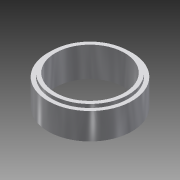
# Autodesk Inventor part: Aluminum Retainer
Saved by Autodesk Inventor 2015 (Build 190159000, 159)
## iProperties
Created: 2016-01-09
Part Number: Aluminum Retainer
Material: Aluminum 6061-AHC
Document SubType Name: Modeling
Designer: Jared
Density: 2.7 g/cm^3
Appearance: Aluminum - Dark
Author: Jared
Autodesk Inventor part; units mm, degrees
ref_plane "YZ Plane" through (0, 0, 0) normal (1, 0, 0) x (0, 1, 0)
ref_plane "XZ Plane" through (0, 0, 0) normal (0, 1, 0) x (-1, 0, 0)
ref_plane "XY Plane" through (0, 0, 0) normal (0, 0, 1) x (1, 0, 0)
sketch "Sketch1" plane through (0, 0, 0) normal (0, 0, 1) x (1, 0, 0)
  arc A0 (-19.4827, -3.287) -> (-19.05, 0) centre (-31.75, 0) ccw
  line L0 (-19.4827, -3.287) -> (-58.7375, -149.7878)
  line L1 (-65.8876, 46.8376) -> (-65.8876, 21.4376)
  line L2 (-65.8876, 21.4376) -> (-71.4375, 21.4376)
  arc A1 (-19.05, 0) -> (-65.8876, 46.8376) centre (-65.8876, 0) ccw
  line L3 (-44.45, 34.1376) -> (-33.8192, 34.1376)
  line L4 (-44.45, 34.1376) -> (-37.3992, -46.4536)
  line L5 (-44.45, 34.1376) -> (0, 34.1376) construction
  line L6 (-37.3992, -46.4536) -> (-31.0492, -46.4536)
  line L7 (-71.4375, 21.4376) -> (-71.4375, 8.7376)
  line L8 (-71.4375, 8.7376) -> (-58.7375, 8.7376)
  line L9 (-58.7375, 8.7376) -> (-52.3875, 8.7376)
  line L10 (-52.3875, 8.7376) -> (-52.3875, -102.3907)
  line L11 (-71.4375, 8.7376) -> (-71.4375, -0.7874)
  line L12 (-71.4375, 8.7376) -> (-61.9125, 8.7376) construction
  line L13 (-71.4375, -0.7874) -> (-58.7375, -0.7874)
  line L14 (-58.7375, -0.7874) -> (-58.7375, -51.5874)
  line L15 (-58.7375, -51.5874) -> (-71.4375, -51.5874)
  line L16 (-71.4375, -0.7874) -> (-65.0875, -0.7874)
  line L17 (-65.0875, -0.7874) -> (-65.0875, -6.731)
  line L18 (-65.0875, -6.731) -> (-71.4375, -6.731)
  line L19 (-71.4375, 21.4376) -> (-71.4375, -0.7874)
  line L20 (-71.4375, -6.731) -> (-71.4375, -51.5874)
  line L21 (-58.7375, -51.5874) -> (-58.7375, -126.0892)
  line L22 (-58.7375, -51.5874) -> (0, -51.5874) construction
  line L23 (-46.0375, -102.3907) -> (-52.3875, -102.3907)
  line L24 (-65.0875, -51.5907) -> (-58.7375, -51.5907)
  line L25 (-58.7375, -149.7878) -> (-61.9125, -161.637)
  line L26 (-58.7375, -149.7878) -> (-34.203, -149.7878) construction
  line L27 (-65.0875, -161.637) -> (-61.9125, -161.637)
  line L28 (-58.7375, -126.0892) -> (-52.3875, -126.0892)
  line L29 (0, 34.1376) -> (0, 0)
  line L30 (-65.0875, -100.6892) -> (-65.0875, -161.637)
  line L31 (-58.7375, -51.5907) -> (-61.9125, -51.5907)
  line L32 (-61.9125, -51.5907) -> (-65.0875, -100.6892)
  dimension "d0" = 19.05
  dimension "d1" = 25.4
  dimension "d2" = 5.5499
  dimension "d3" = 65.8876
  dimension "d4" = 85
  dimension "d5" = 12.7
  dimension "d6" = 46.8376
  dimension "d7" = 12.7
  dimension "d8" = 44.45
  dimension "d9" = 6.35
  dimension "d10" = 105
  dimension "d11" = 12.7
  dimension "d12" = 12.7
  dimension "d13" = 6.35
  dimension "d14" = 9.525
  dimension "d15" = 50.8
  dimension "d16" = 12.7
  dimension "d17" = 6.35
  dimension "d18" = 5.9436
  dimension "d19" = 6.35
  dimension "d20" = 50.8
  dimension "d21" = 6.35
  dimension "d22" = 105
  dimension "d23" = 3.175
  dimension "d24" = 6.35
  dimension "d25" = 60.9478
  dimension "d26" = 3.175
  dimension "d27" = 6.35
  constraints: 67 end point, 14 perpendicular, 9 horizontal, 6 point on line, 5 point on circle, 4 vertical, 3 horizontal alignment, 2 centre point, 2 collinear, 2 midpoint, 1 parallel, 1 tangent, 1 vertical alignment, 1 other
  measures "d0" distance of L29.end A0.end
  measures "d1" distance of L1.start L2.start
  measures "d2" distance of L2.start L7.start
  measures "d3" distance from line of L29.end L1
  measures "d4" angle of L4 L5
  measures "d5" vertical distance of L4.start L1.start
  measures "d6" radius of A1
  measures "d7" radius of A0
  measures "d8" horizontal distance of L29.end L4.start
  measures "d9" distance of L4.end L6.end
  measures "d10" angle of L6 L0
  measures "d11" distance of L7.start L8.start
  measures "d12" distance of L8.start L9.start
  measures "d13" distance of L9.start L9.end
  measures "d14" distance of L8.start L16.start
  measures "d15" distance of L14.start L15.start
  measures "d16" distance of L16.start L14.start
  measures "d17" distance of L16.start L17.start
  measures "d18" distance of L17.start L17.end
  measures "d19" distance of L10.end L23.start
  measures "d20" distance between parallel lines of L23 L24
  measures "d21" distance of L24.start L31.start
  measures "d22" angle of L25 L26
  measures "d23" distance of L27.end L30.end
  measures "d24" distance of L21.end L28.end
  measures "d25" distance of L32.end L30.end
  measures "d26" distance of L31.start L31.end
  measures "d27" distance from line of L21 L32.end
revolve "Revolution1" add sketch "Sketch1" angle 360 about axis through (0, 34.1376, 0) along (0, -1, 0) contours L15 L20 L18 L17 L13 L14
body "Solid1"
